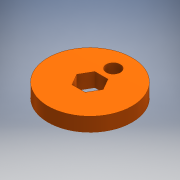
# Autodesk Inventor part: OutputDisk2
Saved by Autodesk Inventor 2016 (Build 200138000, 138)
## iProperties
Created: 2015-12-09
Part Number: OutputDisk2
Material: Generic
Document SubType Name: Modeling
Designer: lk8187
Density: 1 g/cm^3
Appearance: Smooth - Light Orange
Author: lk8187
Autodesk Inventor part; units mm, degrees
ref_plane "YZ Plane" through (0, 0, 0) normal (1, 0, 0) x (0, 1, 0)
ref_plane "XZ Plane" through (0, 0, 0) normal (0, 1, 0) x (-1, 0, 0)
ref_plane "XY Plane" through (0, 0, 0) normal (0, 0, 1) x (1, 0, 0)
sketch "Sketch1" plane through (0, 0, 0) normal (0, 0, 1) x (1, 0, 0)
  circle A0 centre (0, 0) radius 9
  circle A1 centre (0, 5) radius 1.5
  line L0 (1.4145, 2.45) -> (2.829, 0)
  line L1 (2.829, 0) -> (1.4145, -2.45)
  line L2 (1.4145, -2.45) -> (-1.4145, -2.45)
  line L3 (-1.4145, -2.45) -> (-2.829, 0)
  line L4 (-2.829, 0) -> (-1.4145, 2.45)
  line L5 (-1.4145, 2.45) -> (1.4145, 2.45)
  dimension "d0" = 18
  dimension "d1" = 4.9
  dimension "d2" = 5
  dimension "d3" = 3
  constraints: 12 end point, 2 centre point, 2 coincident, 1 horizontal, 1 vertical alignment, 13 other
  measures "d0" diameter of A0
  measures "d1" distance between parallel lines of L2 L5
  measures "d2" distance of point (0, 0) A1.centre
  measures "d3" diameter of A1
extrude "Extrusion1" add sketch "Sketch1" against normal blind 3
body "Solid1"
